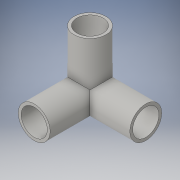
# Autodesk Inventor part: pvc 1in 3 way elbow noah
Saved by Autodesk Inventor 2016 (Build 200138000, 138)
## iProperties
Created: 2017-01-30
Part Number: pvc 1in 3 way elbow noah
Material: Generic
Document SubType Name: Modeling
Designer: Student
Density: 1 g/cm^3
Appearance: Default
Author: Student
Autodesk Inventor part; units mm, degrees
ref_plane "YZ Plane" through (0, 0, 0) normal (1, 0, 0) x (0, 1, 0)
ref_plane "XZ Plane" through (0, 0, 0) normal (0, 1, 0) x (-1, 0, 0)
ref_plane "XY Plane" through (0, 0, 0) normal (0, 0, 1) x (1, 0, 0)
sketch "Sketch1" plane through (0, 0, 0) normal (0, 1, 0) x (-1, 0, 0)
  circle A0 centre (0, 0) radius 20.32
  circle A1 centre (0, 0) radius 16.7005
  dimension "d0" = 40.64
  dimension "d1" = 33.401
  constraints: 2 centre point, 2 coincident
  measures "d0" diameter of A0
  measures "d1" diameter of A1
extrude "Extrusion1" add sketch "Sketch1" along normal blind 71.12
sketch "Sketch2" plane through (0, 0, 0) normal (0, 0, 1) x (1, 0, 0)
  line L0 (-20.32, 0) -> (20.32, 0) projected
  circle A0 centre (0, 0) radius 20.32
  circle A1 centre (0, 0) radius 16.7005
  line L1 (-16.7005, 0) -> (-16.7005, 71.12) projected
  constraints: 2 coincident, 1 centre point, 1 horizontal alignment, 1 tangent, 2 other
extrude "Extrusion2" add sketch "Sketch2" along normal blind 71.12 contours A0 L1 L0 | L0 A1 A0 | L1 A0 L0 A1
sketch "Sketch3" plane through (0, 0, 0) normal (1, 0, 0) x (0, 1, 0)
  line L0 (0, -16.7005) -> (0, 0) projected
  circle A0 centre (0, 0) radius 20.32
  line L1 (-20.32, 0) -> (-20.32, 71.12) projected
  line L2 (0, 0) -> (0, 16.7005) projected
  line L3 (0, 0) -> (-16.7005, 0) projected
  circle A1 centre (0, 0) radius 16.7005
  constraints: 2 coincident, 1 centre point, 1 horizontal alignment, 1 tangent, 2 other
extrude "Extrusion3" add sketch "Sketch3" along normal blind 71.12
sketch "Sketch4" plane through (0, 0, 0) normal (-1, 0, 0) x (0, 0, 1)
  point P0 (0, 0)
body "Solid1"
